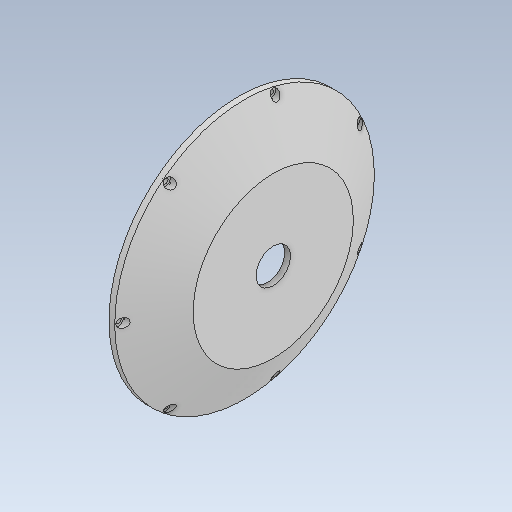
# Autodesk Inventor part: Peça35
Saved by Autodesk Inventor 2021 (Build 250183000, 183)
## iProperties
Category: 41
Created: 2021-07-21
Part Number: Peça35
Material: Genérico
Document SubType Name: Modeling
Designer: Giovanni
Density: 1 g/cm^3
Appearance: Padrão
User Status: 1:8
Author: Giovanni
Keywords: 35
Autodesk Inventor part; units mm, degrees
ref_plane "YZ Plane" through (0, 0, 0) normal (1, 0, 0) x (0, 1, 0)
ref_plane "XZ Plane" through (0, 0, 0) normal (0, 1, 0) x (-1, 0, 0)
ref_plane "XY Plane" through (0, 0, 0) normal (0, 0, 1) x (1, 0, 0)
sketch "Esboço1" plane through (0, 0, 0) normal (0, 0, 1) x (1, 0, 0)
  line L0 (0, 0) -> (60, 0)
  line L1 (0, 208.841) -> (10, 208.841)
  line L2 (10, 208.841) -> (50, 139.559)
  line L3 (50, 139.559) -> (50, 30)
  line L4 (50, 30) -> (60, 30)
  line L5 (0, 208.841) -> (0, 226)
  line L6 (0, 226) -> (10, 226)
  line L7 (10, 226) -> (60, 139.3975)
  line L8 (60, 139.3975) -> (60, 30)
  dimension "d0" = 60
  dimension "d1" = 417.682
  dimension "d2" = 60
  dimension "d3" = 10
  dimension "d4" = 60
  dimension "d5" = 10
  dimension "d6" = 452
  constraints: 18 end point, 3 perpendicular, 3 vertical alignment, 2 horizontal, 1 parallel, 1 vertical
  measures "d0" distance of L0.start L0.end
  measures "d1" diameter of L1 L0
  measures "d2" diameter of L4 L0
  measures "d3" distance of L1.start L1.end
  measures "d4" angle of L2 L1
  measures "d5" distance of L3.end L4.end
  measures "d6" diameter of L6 L0
revolve "Revolução1" add sketch "Esboço1" angle 360 about axis through (0, 0, 0) along (1, 0, 0)
sketch "Esboço2" plane through (60, 0, 0) normal (1, 0, 0) x (0, 0, -1)
  circle A0 centre (0, 0) radius 139.3975 projected
  point P0 (-217, 0)
  dimension "d8" = 217
  constraints: 1 horizontal alignment
  measures "d8" distance of point (-217, 0) A0.centre
hole "Furo1" at (60, 0, 217) direction (-1, 0, 0) diameter 8.5 end through all counterbore diameter 16 counterbore depth 52 clearance for "Socket Head Cap Screw DIN EN ISO 4762" size "M8" standard "DIN"
pattern_circular "Padrão circular1" count 7 over 360 about axis through (55, 0, 0) along (1, 0, 0) of "Furo1"
